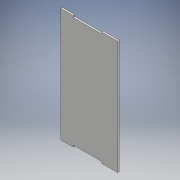
# Autodesk Inventor part: Piso
Saved by Autodesk Inventor 2018 (Build 220112000, 112)
## iProperties
Created: 2020-03-11
Part Number: Piso
Material: Genérico
Document SubType Name: Modeling
Designer: joser
Density: 1 g/cm^3
Appearance: Valor por defecto
Author: joser
Autodesk Inventor part; units mm, degrees
ref_plane "YZ Plane" through (0, 0, 0) normal (1, 0, 0) x (0, 1, 0)
ref_plane "XZ Plane" through (0, 0, 0) normal (0, 1, 0) x (-1, 0, 0)
ref_plane "XY Plane" through (0, 0, 0) normal (0, 0, 1) x (1, 0, 0)
sketch "Boceto1" plane through (0, 0, 0) normal (0, 1, 0) x (-1, 0, 0)
  line L0 (50, 100) -> (50, -100)
  line L1 (-50, 100) -> (50, -100) construction
  line L2 (50, 100) -> (-50, -100) construction
  line L3 (28, 100) -> (28, 97)
  line L4 (28, 97) -> (-22, 97)
  line L5 (-22, 97) -> (-22, 100)
  line L6 (-50, 100) -> (-22, 100)
  line L7 (28, 100) -> (50, 100)
  line L8 (28, -100) -> (28, -97)
  line L9 (28, -97) -> (-22, -97)
  line L10 (-22, -97) -> (-22, -100)
  line L11 (50, -100) -> (28, -100)
  line L12 (-22, -100) -> (-50, -100)
  line L13 (-50, -100) -> (-50, 100)
  point P0 (0, 0)
  dimension "d0" = 100
  dimension "d1" = 200
  dimension "d4" = 3
  dimension "d5" = 50
  dimension "d7" = 3
  dimension "d8" = 50
  dimension "d12" = 28
  constraints: 28 end point, 8 perpendicular, 5 parallel, 3 collinear, 2 horizontal, 2 midpoint, 2 vertical
  measures "d0" distance of L0.end L2.end
  measures "d1" distance of L0.start L0.end
  measures "d4" distance of L3.start L3.end
  measures "d5" distance of L3.end L4.end
  measures "d7" distance of L8.start L8.end
  measures "d8" distance of L8.end L9.end
  measures "d12" distance between parallel lines of L13 L5
extrude "Extrusión1" add sketch "Boceto1" along normal blind 3
